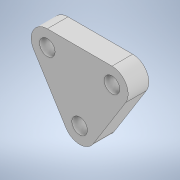
# Autodesk Inventor part: f3
Saved by Autodesk Inventor 2020 (Build 240168000, 168)
## iProperties
Created: 2020-11-09
Part Number: f3
Material: Generic
Document SubType Name: Modeling
Designer: alnwlsn
Density: 1 g/cm^3
Appearance: Default
Author: alnwlsn
Autodesk Inventor part; units mm, degrees
ref_plane "YZ Plane" through (0, 0, 0) normal (1, 0, 0) x (0, 1, 0)
ref_plane "XZ Plane" through (0, 0, 0) normal (0, 1, 0) x (-1, 0, 0)
ref_plane "XY Plane" through (0, 0, 0) normal (0, 0, 1) x (1, 0, 0)
sketch "Sketch1" plane through (0, 0, 0) normal (0, 0, 1) x (1, 0, 0)
  circle A0 centre (0, 0) radius 1.25
  circle A1 centre (5, 0) radius 1.25
  line L0 (0, 0) -> (5, 0)
  circle A2 centre (2.5, -4) radius 1.25
  line L1 (-1.06, -0.6625) -> (1.44, -4.6625)
  line L2 (3.56, -4.6625) -> (6.06, -0.6625)
  line L3 (5, 1.25) -> (0, 1.25)
  circle A3 centre (0, 0) radius 0.6
  circle A4 centre (5, 0) radius 0.6
  circle A5 centre (2.5, -4) radius 0.6
  dimension "d0" = 5
  dimension "d1" = 2.5
  dimension "d2" = 4
  dimension "d3" = 1.2
  constraints: 8 end point, 6 centre point, 6 point on circle, 6 tangent, 4 equal radius, 3 coincident, 1 concentric, 1 equal length, 1 horizontal, 1 point on line
  measures "d0" distance of L0.end point (0, 0)
  measures "d1" diameter of A1
  measures "d2" distance from line of L0 A2.centre
  measures "d3" diameter of A4
extrude "Extrusion1" add sketch "Sketch1" along normal blind 1.6
body "Solid1"
